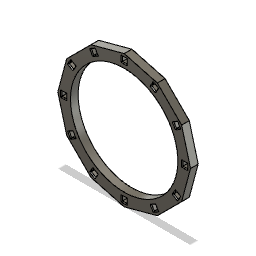
4in_PVC_DWV_Fitting v2 (Autodesk Fusion 360 archive; units mm, degrees)
design "4_Magnetic_Face"
Autodesk Fusion 360 part; units mm, degrees
sketch "Sketch1" plane through (0, 0, 0) normal (0, 0, 1) x (1, 0, 0)
  circle A0 centre (0, 0) radius 50.8
  circle A1 centre (0, 0) radius 49
  dimension "d1" = 101.6
  dimension "d2" = 1.8
  constraint coincident A0.centre A1.centre
  constraint concentric A0 A1
  measures "d1" diameter of A0
  measures "d2" distance of A0 A1
extrude "Extrude1" add sketch "Sketch1" along normal blind 7
sketch "Sketch2" plane through (0, 0, 7) normal (0, 0, 1) x (1, 0, 0)
  circle A0 centre (0, 0) radius 49
  circle A1 centre (0, 0) radius 50.8
  line L0 (-30.275, -52.4378) -> (0, -60.55)
  line L1 (0, -60.55) -> (30.275, -52.4378)
  line L2 (30.275, -52.4378) -> (52.4378, -30.275)
  line L3 (52.4378, -30.275) -> (60.55, 0)
  line L4 (60.55, 0) -> (52.4378, 30.275)
  line L5 (52.4378, 30.275) -> (30.275, 52.4378)
  line L6 (30.275, 52.4378) -> (0, 60.55)
  line L7 (0, 60.55) -> (-30.275, 52.4378)
  line L8 (-30.275, 52.4378) -> (-52.4378, 30.275)
  line L9 (-52.4378, 30.275) -> (-60.55, 0)
  line L10 (-60.55, 0) -> (-52.4378, -30.275)
  line L11 (-52.4378, -30.275) -> (-30.275, -52.4378)
  line L12 (-2.375, 52.8) -> (2.375, 52.8)
  line L13 (2.375, 52.8) -> (2.375, 57.55)
  line L14 (2.375, 57.55) -> (-2.375, 57.55)
  line L15 (-2.375, 57.55) -> (-2.375, 52.8)
  line L16 (-2.375, 52.8) -> (2.375, 57.55) construction
  line L17 (2.375, 52.8) -> (-2.375, 57.55) construction
  point P0 (0, 55.175)
  point P1 (0, 52.8)
  point P2 (0, 50.8)
  dimension "d5" = 4.75
  dimension "d6" = 3
  dimension "d7" = 2
  constraint coincident A0.centre A1.centre
  constraint vertical L6.end A0.centre
  constraint horizontal L12
  constraint perpendicular L12 L13
  constraint parallel L12 L14
  constraint parallel L13 L15
  constraint coincident L16 P0
  constraint coincident L17 P0
  constraint equal L12 L15
  constraint vertical A0.centre P0
  constraint midpoint L12 P1
  constraint coincident A1 P2
  constraint vertical A0.centre P2
  measures "d5" distance of L12 L14
  measures "d6" distance of L6.end L14
  measures "d7" distance of P1 P2
extrude "Extrude2" add sketch "Sketch2" against normal up to surface (7 mm away) contours L0 L1 L2 L3 L4 L5 L6 L7 L8 L9 L10 L11 | L12 L13 L14 L15
extrude "Extrude3" cut sketch "Sketch2" against normal blind 5.5 contours L12 L13 L14 L15
chamfer "Chamfer1" distance 0.5 angle 60 4 edges at (2.375, 55.175, 7) (0, 57.55, 7) (-2.375, 55.175, 7) (0, 52.8, 7) measured on face at (-53.2703, 14.906, 7) measured on face at (-53.2703, 14.906, 7) measured on face at (-53.2703, 14.906, 7) measured on face at (-53.2703, 14.906, 7)
pattern_circular "C-Pattern1" count 12 over 360 about axis through (0, 0, 1.75) along (0, 0, 1) of "Extrude3", "Chamfer1"
